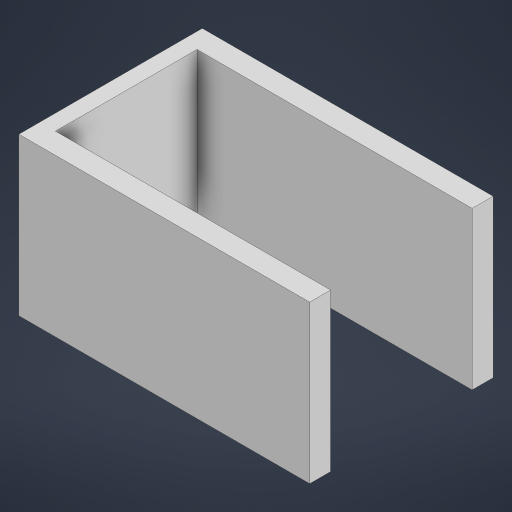
# Autodesk Inventor part: soporte_brazo
Saved by Autodesk Inventor 2023.1 (Build 271208000, 208)
## iProperties
Created: 2022-11-07
Part Number: soporte_brazo
Material: Generic
Document SubType Name: Modeling
Designer: amtat
Density: 1 g/cm^3
Appearance: Default
Author: amtat
Autodesk Inventor part; units mm, degrees
ref_plane "YZ Plane" through (0, 0, 0) normal (1, 0, 0) x (0, 1, 0)
ref_plane "XZ Plane" through (0, 0, 0) normal (0, 1, 0) x (-1, 0, 0)
ref_plane "XY Plane" through (0, 0, 0) normal (0, 0, 1) x (1, 0, 0)
sketch "Sketch1" plane through (0, 0, 0) normal (1, 0, 0) x (0, 1, 0)
  line L0 (0, 0) -> (0, -31)
  line L1 (0, -31) -> (30, -31)
  line L2 (30, -31) -> (30, 0)
  line L3 (30, 0) -> (0, 0)
  line L4 (0, -31) -> (0, -33)
  line L5 (0, -33) -> (30, -33)
  line L6 (30, -33) -> (30, -31)
  line L7 (30, 0) -> (30, 2)
  line L8 (30, 2) -> (0, 2)
  line L9 (0, 2) -> (0, 0)
  dimension "d0" = 31
  dimension "d1" = 30
  dimension "d2" = 31
  dimension "d5" = 2
  dimension "d6" = 2
  constraints: 20 end point, 4 perpendicular, 2 point on line, 2 vertical, 1 collinear, 1 horizontal
  measures "d0" distance of L0.start L0.end
  measures "d1" distance of L0.end L1.end
  measures "d2" distance of L1.end L2.end
  measures "d5" distance of L0.end L4.end
  measures "d6" distance of L2.end L7.end
extrude "Extrusion2" add sketch "Sketch1" along normal blind 3
sketch "Sketch2" plane through (3, 0, 0) normal (1, 0, 0) x (0, 0, -1)
  line L0 (33, 30) -> (-2, 30) projected
  line L1 (-2, 30) -> (2, 30)
  line L2 (2, 30) -> (2, 0)
  line L3 (-2, 0) -> (33, 0) projected
  line L4 (33, 0) -> (33, 30) projected
  line L5 (33, 30) -> (-2, 30) projected
  line L6 (-2, 30) -> (-2, 0) projected
  line L7 (-2, 0) -> (33, 0) projected
  line L8 (33, 0) -> (33, 30) projected
  line L9 (33, 30) -> (29, 30)
  line L10 (29, 30) -> (29, 0)
  point P0 (0, 0)
  dimension "d9" = 4
  dimension "d10" = 4
  constraints: 8 end point, 4 point on line, 2 perpendicular
  measures "d9" distance of L0.end L1.end
  measures "d10" distance of L0.start L9.end
extrude "Extrusion3" add sketch "Sketch2" along normal blind 52.5 contours L4 L3 L10 L0 | L2 L3 L6 L0
body "Solid2"
